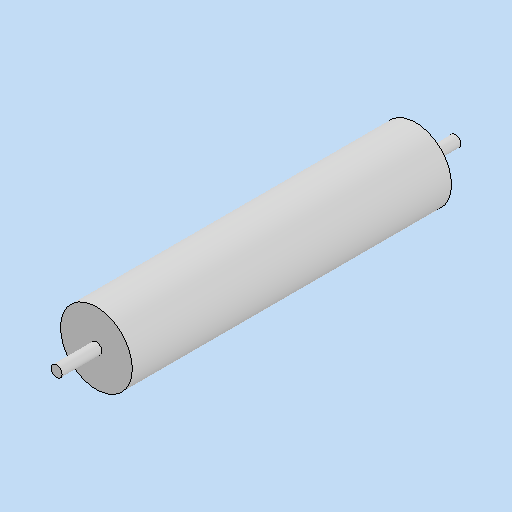
# Autodesk Inventor part: 15kOhmResistor
Saved by Autodesk Inventor 2025 (Build 290162000, 162)
## iProperties
Created: 2025-03-14
Part Number: 15kOhmResistor
Material: Generic
Document SubType Name: Modeling
Designer: kuzmin
Density: 1 g/cm^3
Appearance: Default
Author: kuzmin
Autodesk Inventor part; units mm, degrees
ref_plane "YZ Plane" through (0, 0, 0) normal (1, 0, 0) x (0, 1, 0)
ref_plane "XZ Plane" through (0, 0, 0) normal (0, 1, 0) x (-1, 0, 0)
ref_plane "XY Plane" through (0, 0, 0) normal (0, 0, 1) x (1, 0, 0)
sketch "Sketch1" plane through (0, 0, 0) normal (0, 1, 0) x (-1, 0, 0)
  line L0 (0, 25) -> (0, -25)
  line L1 (0, 25) -> (0.7, 25)
  line L2 (0.7, 25) -> (0.7, 20)
  line L3 (0.7, 20) -> (4.5, 20)
  line L4 (4.5, 20) -> (4.5, -20)
  line L5 (4.5, -20) -> (0.7, -20)
  line L6 (0.7, -20) -> (0.7, -25)
  line L7 (0.7, -25) -> (0, -25)
  point P0 (0, 0)
  point P1 (0, 0)
  dimension "d0" = 9
  dimension "d1" = 1.4
  dimension "d2" = 5
  dimension "d3" = 40
  constraints: 16 end point, 5 perpendicular, 2 point on line, 1 coincident, 1 collinear, 1 horizontal, 1 midpoint, 1 vertical
  measures "d0" diameter of L4 L0
  measures "d1" diameter of L2 L0
  measures "d2" distance of L1.end L2.end
  measures "d3" distance of L3.end L4.end
revolve "Revolution1" add sketch "Sketch1" angle 360 about axis through (0, 0, 25) along (0, 0, -1)
body "Solid1"
